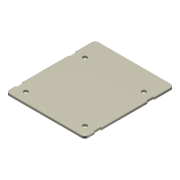
# Autodesk Inventor part: SLIPRING_SRG-1-6G_
Saved by Autodesk Inventor 2011 SP1 (Build 150282100, 282)
## iProperties
Created: 2012-05-23
Part Number: SLIPRING_SRG-1-6G_
Document SubType Name: Modeling
Designer: arihon
Density: 1 g/cm^3
Author: arihon
Autodesk Inventor part; units mm, degrees
ref_plane "YZ Plane" through (0, 0, 0) normal (1, 0, 0) x (0, 1, 0)
ref_plane "XZ Plane" through (0, 0, 0) normal (0, 1, 0) x (-1, 0, 0)
ref_plane "XY Plane" through (0, 0, 0) normal (0, 0, 1) x (1, 0, 0)
sketch "スケッチ1" plane through (0, 0, 0) normal (0, 0, 1) x (1, 0, 0)
  circle A0 centre (13.0815, -13.0815) radius 1
  circle A1 centre (-13.0815, 13.0815) radius 1
  circle A2 centre (13.0815, 13.0815) radius 1
  line L0 (-17.5, -17.5) -> (17.5, -17.5)
  line L1 (17.5, -17.5) -> (17.5, -13.2)
  line L2 (17.5, 22) -> (-17.5, 22)
  line L3 (-17.5, 22) -> (-17.5, 13.2505)
  line L4 (-17.0382, 13.2505) -> (-17.5, 13.2505)
  line L5 (-17.5, 13.2505) -> (-17.5, 13.2)
  line L6 (-17.5, 10.2) -> (-17.0382, 10.2)
  line L7 (-17.0382, 10.2) -> (-17.0382, 13.2505)
  line L8 (-17, -10.2) -> (-17.5, -10.2)
  line L9 (-17.5, -10.2) -> (-17.5, -13.2)
  line L10 (-17.5, -13.2) -> (-17, -13.2)
  line L11 (-17, -13.2) -> (-17, -10.2)
  line L12 (17.5, -10.2) -> (17, -10.2)
  line L13 (17, -10.2) -> (17, -13.2)
  line L14 (17, -13.2) -> (17.5, -13.2)
  line L15 (17.5, -13.2) -> (17.5, -10.2)
  line L16 (17.5, 13.2) -> (17, 13.2)
  line L17 (17, 13.2) -> (17, 10.2)
  line L18 (17, 10.2) -> (17.5, 10.2)
  line L19 (17.5, 10.2) -> (17.5, 13.2)
  line L20 (17, 13.2) -> (17.5, 13.2)
  line L21 (17.5, 13.2) -> (17.5, 22)
  line L22 (17.5, 10.2) -> (17.5, 13.2)
  line L23 (17.5, -10.2) -> (17.5, 10.2)
  line L24 (17.5, -13.2) -> (17.5, -10.2)
  line L25 (-17.5, -13.2) -> (-17.5, -17.5)
  line L26 (-17.5, -10.2) -> (-17.5, -13.2)
  line L27 (-17.5, 13.2505) -> (-17.5, 13.2)
  line L28 (-17.5, 13.2) -> (-17.5, 10.2)
  line L29 (-17.5, 10.2) -> (-17.5, -10.2)
  line L30 (-17.5, 13.2) -> (-17.5, 10.2)
  circle A3 centre (-13.0815, 13.0815) radius 1
  circle A4 centre (13.0815, 13.0815) radius 1
  circle A5 centre (-13.0815, -13.0815) radius 1
  circle A6 centre (13.0815, -13.0815) radius 1
  circle A7 centre (-13.0815, -13.0815) radius 1
  point P0 (0, 0)
  point P1 (0, 0)
  dimension "d0" = 39.5
  dimension "d1" = 2
  constraints: 63 end point, 40 parallel, 10 perpendicular, 8 centre point, 5 horizontal, 4 coincident, 3 concentric, 2 point on line
  measures "d0" distance of L2.end L0.start
  measures "d1" diameter of A5
extrude "押し出し1" add sketch "スケッチ1" along normal blind 1 contours L25 L10 L11 L8 L29 L6 L7 L4 L3 L2 L21 L16 L17 L18 L23 L12 L13 L14 L1 L0
fillet "フィレット1" radius 1.5 4 edges at (-17.5, -17.5, 0.5) (-17.5, 22, 0.5) (17.5, 22, 0.5) (17.5, -17.5, 0.5)
